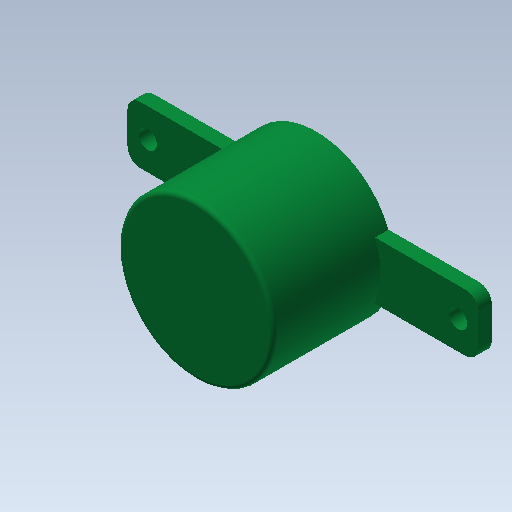
# Autodesk Inventor part: HEDR-5420-ES214
Saved by Autodesk Inventor 2020.3 (Build 243373000, 373)
## iProperties
RuleStatus: InUse
AfterDocSave0: file://Part Number Cleaner
Created: 2014-11-19
Material: FR4
Vendor: AVAGO / DIGI-KEY
Document SubType Name: Modeling
Designer: ARNOLDJ
Density: 1.1 g/cm^3
Description: ENCODER MODULE 200CPR 5MM
Project: P-209503
Mass: 8.69372 g
Surface Area: 27.2643 cm^2
Volume: 7.90338 cm^3
Appearance: Green (Flat)
LAB/DEPT: CUI (LAB)
REQUESTING SCIENTIST: KONG, LINGJIE
SURFACE ROUGHNESS: N/A
DESIGN DEPARTMENT: HHMI: JFRC - ID&F
SPECIAL FINISH: NONE
ALTERED ITEM PART NUMBER: N/A
ALTERED ITEM VENDOR: N/A
ALTERED ITEM DESCRIPTION: N/A
Revision Number: 0
Autodesk Inventor part; units mm, degrees
ref_plane "YZ Plane" through (0, 0, 0) normal (1, 0, 0) x (0, 1, 0)
ref_plane "XZ Plane" through (0, 0, 0) normal (0, 1, 0) x (-1, 0, 0)
ref_plane "XY Plane" through (0, 0, 0) normal (0, 0, 1) x (1, 0, 0)
sketch "Sketch1" plane through (0, 0, 0) normal (0, 0, 1) x (1, 0, 0)
  circle A0 centre (0, 0) radius 11.5
  line L0 (-26, 4.25) -> (26, 4.25)
  line L1 (26, 4.25) -> (26, -4.25)
  line L2 (26, -4.25) -> (-26, -4.25)
  line L3 (-26, -4.25) -> (-26, 4.25)
  point P0 (-26, 0)
  point P1 (0, 4.25)
  dimension "d0" = 23
  dimension "d1" = 52
  dimension "d2" = 8.5
  constraints: 8 end point, 2 midpoint, 2 parallel, 1 centre point, 1 coincident, 1 horizontal, 1 horizontal alignment, 1 perpendicular, 1 vertical alignment
  measures "d0" diameter of A0
  measures "d1" distance of L0.start L0.end
  measures "d2" distance of L0.end L1.end
extrude "Extrusion1" add sketch "Sketch1" along normal blind 2 contours A0 L2 L0 | A0 L0 L1 L2 | A0 L2 L3 L0
extrude "Extrusion2" add sketch "Sketch1" along normal blind 17.9 contours A0 L2 L0 | L0 A0 | A0 L2
sketch "Sketch2" plane through (0, 0, 0) normal (0, 0, 1) x (1, 0, 0)
  line L0 (-27.9259, 0) -> (33.5172, 0) construction
  point P0 (0, 0)
  point P1 (-23, 0)
  point P2 (23, 0)
  dimension "d7" = 0
  dimension "d8" = 23
  dimension "d9" = 23
  constraints: 2 end point, 2 point on line, 1 horizontal
  measures "d7" distance from line of L0 point (0, 0)
  measures "d8" distance of point (0, 0) point (-23, 0)
  measures "d9" distance of point (23, 0) point (0, 0)
hole "Hole1" at (-23, 0, 0) at (23, 0, 0) direction (0, 0, 1) diameter 2.7178 end through all
fillet "Fillet1" radius 1.905 4 edges at (-26, -4.25, 1) (26, -4.25, 1) (26, 4.25, 1) (-26, 4.25, 1)
fillet "Fillet2" radius 0.635 1 edges at (-11.5, 0, 17.9)
hole "Hole2" at (0, 0, 0) direction (0, 0, 1) diameter 8.89 depth 12.7 tip angle 118
body "Solid1"
